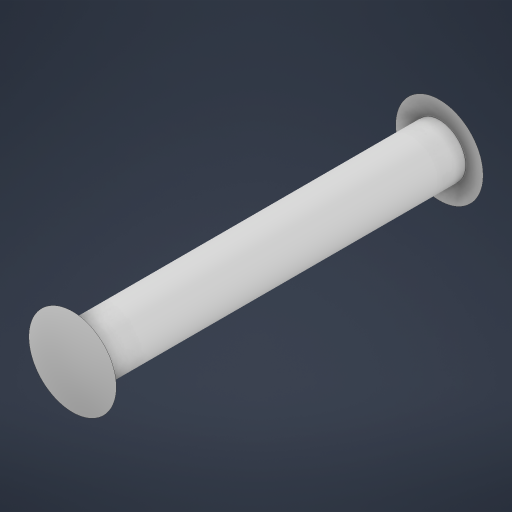
# Autodesk Inventor part: Część5
Saved by Autodesk Inventor 2023 (Build 270158000, 158)
## iProperties
Created: 2023-05-18
Part Number: Część5
Material: Ogólny
Document SubType Name: Modeling
Designer: Adam
Density: 1 g/cm^3
Appearance: Domyślna
Author: Adam
Autodesk Inventor part; units mm, degrees
ref_plane "YZ Plane" through (0, 0, 0) normal (1, 0, 0) x (0, 1, 0)
ref_plane "XZ Plane" through (0, 0, 0) normal (0, 1, 0) x (-1, 0, 0)
ref_plane "XY Plane" through (0, 0, 0) normal (0, 0, 1) x (1, 0, 0)
sketch "Szkic1" plane through (0, 0, 0) normal (0, 1, 0) x (-1, 0, 0)
  line L0 (1, 10.5) -> (0, 10.5)
  line L1 (0, 10.5) -> (0, -10.5)
  line L2 (0, -10.5) -> (1, -10.5)
  arc A0 (1, 10.5) -> (-4, 10.5) centre (-1.5, 4.5) ccw
  arc A1 (-4, -10.5) -> (1, -10.5) centre (-1.5, -4.5) ccw
  line L3 (-1.5, -4.5) -> (-1.5, 4.5)
  line L4 (-1.5, 11) -> (-1.5, -11)
  point P0 (0, 0)
  point P1 (0, 0)
  dimension "d0" = 1
  dimension "d4" = 5
  dimension "d5" = 1
  constraints: 10 end point, 6 point on circle, 2 centre point, 1 coincident, 1 horizontal, 1 midpoint, 1 vertical
  measures "d0" distance of L0.start L0.end
  measures "d4" distance of L0.start A0.end
  measures "d5" distance of L1.end L2.end
revolve "Obrót1" add sketch "Szkic1" angle 360 about axis through (1.5, 0, 11) along (0, 0, -1)
